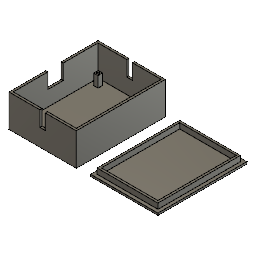
Circuit_Housing 3 (Autodesk Fusion 360 design; units mm, degrees)
Autodesk Fusion 360 part; units mm, degrees
sketch "Sketch1" plane through (0, 0, 0) normal (0, 1, 0) x (1, 0, 0)
  line L0 (-31, -41) -> (31, -41)
  line L1 (31, -41) -> (31, 41)
  line L2 (31, 41) -> (-31, 41)
  line L3 (-31, 41) -> (-31, -41)
  line L4 (-31, -41) -> (31, 41) construction
  line L5 (31, -41) -> (-31, 41) construction
  dimension "d1" = 62
  dimension "d2" = 82
  constraint horizontal L0
  constraint perpendicular L0 L1
  constraint parallel L0 L2
  constraint parallel L1 L3
  constraint coincident L4 origin
  constraint coincident L5 origin
  measures "d1" distance of L1.end L2.end
  measures "d2" distance of L0.end L1.end
extrude "Extrude1" add sketch "Sketch1" along normal blind 30 thin wall 2 inside makes body 1
sketch "Sketch4" plane through (0, 0, 0) normal (0, 1, 0) x (1, 0, 0)
  line L0 (-29, -39) -> (29, -39)
  line L1 (29, -39) -> (29, 39)
  line L2 (29, 39) -> (-29, 39)
  line L3 (-29, 39) -> (-29, -39)
  line L4 (-29, -39) -> (29, 39) construction
  line L5 (29, -39) -> (-29, 39) construction
  dimension "d8" = 58
  dimension "d9" = 78
  constraint horizontal L0
  constraint perpendicular L0 L1
  constraint parallel L0 L2
  constraint parallel L1 L3
  constraint coincident L4 origin
  constraint coincident L5 origin
  measures "d8" distance of L1.end L2.end
  measures "d9" distance of L0.end L1.end
extrude "Extrude2" add sketch "Sketch4" along normal blind 2 bodies 1
sketch "Sketch5" plane through (0, 2, 0) normal (0, 1, 0) x (-1, 0, 0)
  line L0 (29, -39) -> (29, 39)
  line L1 (29, 39) -> (-29, 39)
  line L2 (-29, 39) -> (-29, -39)
  line L3 (-29, -39) -> (29, -39)
  line L4 (25, -35) -> (21, -35)
  line L5 (21, -35) -> (21, -31)
  line L6 (21, -31) -> (25, -31)
  line L7 (25, -31) -> (25, -35)
  line L8 (25, -35) -> (21, -31) construction
  line L9 (21, -35) -> (25, -31) construction
  circle A0 centre (23, -33) radius 1.1
  line L10 (-25, -35) -> (-21, -35)
  line L11 (-21, -35) -> (-21, -31)
  line L12 (-21, -31) -> (-25, -31)
  line L13 (-25, -31) -> (-25, -35)
  line L14 (-25, 35) -> (-21, 35)
  line L15 (-21, 35) -> (-21, 31)
  line L16 (-21, 31) -> (-25, 31)
  line L17 (-25, 31) -> (-25, 35)
  line L18 (25, 35) -> (21, 35)
  line L19 (21, 35) -> (21, 31)
  line L20 (21, 31) -> (25, 31)
  line L21 (25, 31) -> (25, 35)
  circle A1 centre (-23, -33) radius 1.1
  circle A2 centre (23, 33) radius 1.1
  circle A3 centre (-23, 33) radius 1.1
  point P0 (23, -33)
  dimension "d14" = 4
  dimension "d15" = 4
  dimension "d16" = 2.2
  dimension "d17" = 4
  dimension "d18" = 4
  dimension "d19" = 4
  dimension "d20" = 4
  dimension "d21" = 4
  dimension "d22" = 4
  dimension "d23" = 2.2
  dimension "d24" = 2.2
  dimension "d25" = 2.2
  constraint horizontal L4
  constraint perpendicular L4 L5
  constraint parallel L4 L6
  constraint parallel L5 L7
  constraint coincident L8 P0
  constraint coincident L9 P0
  constraint coincident P0 A0.centre
  constraint horizontal L10
  constraint vertical L11
  constraint horizontal L12
  constraint vertical L13
  constraint horizontal L14
  constraint vertical L15
  constraint horizontal L16
  constraint vertical L17
  constraint horizontal L18
  constraint vertical L19
  constraint horizontal L20
  constraint vertical L21
  measures "d14" distance of L5.end L6.end
  measures "d15" distance of L4.end L5.end
  measures "d16" diameter of A0
  measures "d17" distance of L10.start L10.end
  measures "d18" distance of L10.start L12.end
  measures "d19" distance of L14.start L14.end
  measures "d20" distance of L14.start L16.end
  measures "d21" distance of L18.start L18.end
  measures "d22" distance of L18.start L20.end
  measures "d23" diameter of A1
  measures "d24" diameter of A2
  measures "d25" diameter of A3
extrude "Extrude3" add sketch "Sketch5" along normal blind 10 separate body contours L4 L5 L6 L7 | L10 L11 L12 L13 | L14 L15 L16 L17 | L18 L19 L20 L21 makes body 2 at (21.9014, 8.6667, -33.0548) makes body 3 at (21.9014, 8.6667, 32.9452) makes body 4 at (-24.0986, 8.6667, -33.0548) makes body 5 at (-24.0986, 8.6667, 32.9452)
sketch "Sketch6" plane through (0, 0, 41) normal (0, 0, 1) x (1, 0, 0)
  line L0 (-31, 0) -> (31, 0)
  line L1 (31, 0) -> (31, 30)
  line L2 (31, 30) -> (-31, 30)
  line L3 (-31, 30) -> (-31, 0)
  line L4 (-2.5, 16) -> (2.5, 16)
  line L5 (2.5, 16) -> (2.5, 30)
  line L6 (2.5, 30) -> (-2.5, 30)
  line L7 (-2.5, 30) -> (-2.5, 16)
  line L8 (-2.5, 16) -> (2.5, 30) construction
  line L9 (2.5, 16) -> (-2.5, 30) construction
  point P0 (0, 23)
  dimension "d28" = 5
  dimension "d29" = 14
  constraint horizontal L4
  constraint perpendicular L4 L5
  constraint parallel L4 L6
  constraint parallel L5 L7
  constraint coincident L8 P0
  constraint coincident L9 P0
  measures "d28" distance of L5.end L6.end
  measures "d29" distance of L4.end L5.end
extrude "Extrude4" cut sketch "Sketch6" against normal blind 85 contours L2 L4 L5 L6 L7 bodies 1
sketch "Sketch8" plane through (-31, 0, 0) normal (-1, 0, 0) x (0, 0, 1)
  line L0 (-41, 0) -> (41, 0)
  line L1 (41, 0) -> (41, 30)
  line L2 (41, 30) -> (-41, 30)
  line L3 (-41, 30) -> (-41, 0)
  line L4 (7, 30) -> (-7, 30)
  line L5 (-7, 30) -> (-7, 16)
  line L6 (-7, 16) -> (7, 16)
  line L7 (7, 16) -> (7, 30)
  line L8 (7, 30) -> (-7, 16) construction
  line L9 (-7, 30) -> (7, 16) construction
  point P0 (0, 23)
  dimension "d36" = 14
  dimension "d37" = 14
  constraint horizontal L4
  constraint perpendicular L4 L5
  constraint parallel L4 L6
  constraint parallel L5 L7
  constraint coincident L8 P0
  constraint coincident L9 P0
  measures "d36" distance of L5.end L6.end
  measures "d37" distance of L4.end L5.end
extrude "Extrude6" cut sketch "Sketch8" against normal blind 2 contours L2 L4 L5 L6 L7 bodies 1
sketch "Sketch12" plane through (0, 0, 0) normal (0, 1, 0) x (1, 0, 0)
  line L0 (44, -41) -> (106, -41)
  line L1 (106, -41) -> (106, 41)
  line L2 (106, 41) -> (44, 41)
  line L3 (44, 41) -> (44, -41)
  line L4 (44, -41) -> (106, 41) construction
  line L5 (106, -41) -> (44, 41) construction
  point P0 (75, 0)
  dimension "d52" = 62
  dimension "d53" = 82
  constraint horizontal L0
  constraint perpendicular L0 L1
  constraint parallel L0 L2
  constraint parallel L1 L3
  constraint coincident L4 P0
  constraint coincident L5 P0
  measures "d52" distance of L1.end L2.end
  measures "d53" distance of L0.end L1.end
extrude "Extrude8" add sketch "Sketch12" along normal blind 2 separate body makes body 6
sketch "Sketch13" plane through (0, 2, 0) normal (0, 1, 0) x (-1, 0, 0)
  line L0 (-44, -41) -> (-44, 41)
  line L1 (-44, 41) -> (-106, 41)
  line L2 (-106, 41) -> (-106, -41)
  line L3 (-106, -41) -> (-44, -41)
  line L4 (-47, 38) -> (-103, 38)
  line L5 (-103, 38) -> (-103, -38)
  line L6 (-103, -38) -> (-47, -38)
  line L7 (-47, -38) -> (-47, 38)
  line L8 (-47, 38) -> (-103, -38) construction
  line L9 (-103, 38) -> (-47, -38) construction
  point P0 (-75, 0)
  dimension "d56" = 56
  dimension "d57" = 76
  constraint horizontal L4
  constraint perpendicular L4 L5
  constraint parallel L4 L6
  constraint parallel L5 L7
  constraint coincident L8 P0
  constraint coincident L9 P0
  measures "d56" distance of L5.end L6.end
  measures "d57" distance of L4.end L5.end
extrude "Extrude9" add sketch "Sketch13" along normal blind 5 thin wall 2 inside contours L4 L5 L6 L7 bodies 6
